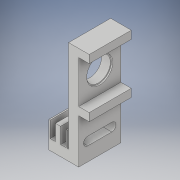
# Autodesk Inventor part: RotateLimitSwitchHolder
Saved by Autodesk Inventor 2018.3 (Build 223284000, 284)
## iProperties
Created: 2019-09-02
Part Number: RotateLimitSwitchHolder
Material: Generic
Document SubType Name: Modeling
Designer: Srinity
Density: 1 g/cm^3
Appearance: Default
Author: Srinity
Autodesk Inventor part; units mm, degrees
ref_plane "YZ Plane" through (0, 0, 0) normal (1, 0, 0) x (0, 1, 0)
ref_plane "XZ Plane" through (0, 0, 0) normal (0, 1, 0) x (-1, 0, 0)
ref_plane "XY Plane" through (0, 0, 0) normal (0, 0, 1) x (1, 0, 0)
sketch "Sketch1" plane through (0, 0, 0) normal (0, 0, 1) x (1, 0, 0)
  line L0 (10.0241, 19.7036) -> (11.6941, 19.7036)
  line L1 (11.6941, 19.7036) -> (11.6941, -12.0464)
  line L2 (11.6941, -12.0464) -> (10.0241, -12.0464)
  line L3 (10.0241, -12.0464) -> (10.0241, 19.7036)
  line L4 (11.6941, -5.6964) -> (18.1941, -5.6964)
  line L5 (18.1941, -5.6964) -> (18.1941, -12.0464)
  line L6 (18.1941, -12.0464) -> (11.6941, -12.0464)
  line L7 (11.6941, -12.0464) -> (11.6941, -5.6964)
  line L8 (18.1941, 19.7036) -> (24.3941, 19.7036)
  line L9 (24.3941, 19.7036) -> (24.3941, -12.0464)
  line L10 (24.3941, -12.0464) -> (18.1941, -12.0464)
  line L11 (18.1941, -12.0464) -> (18.1941, 19.7036)
  line L12 (24.3941, -5.6964) -> (30.8941, -5.6964)
  line L13 (30.8941, -5.6964) -> (30.8941, -12.0464)
  line L14 (30.8941, -12.0464) -> (24.3941, -12.0464)
  line L15 (24.3941, -12.0464) -> (24.3941, -5.6964)
  line L16 (30.8941, 19.7036) -> (32.5641, 19.7036)
  line L17 (32.5641, 19.7036) -> (32.5641, -12.0464)
  line L18 (32.5641, -12.0464) -> (30.8941, -12.0464)
  line L19 (30.8941, -12.0464) -> (30.8941, 19.7036)
  line L20 (14.9441, -5.6964) -> (14.9441, -6.8027)
  line L21 (27.6441, -5.6964) -> (27.6441, -11.0357)
  line L22 (10.0241, 0.6536) -> (32.5641, 0.6536)
  line L23 (32.5641, 0.6536) -> (32.5641, -12.0464)
  line L24 (32.5641, -12.0464) -> (10.0241, -12.0464)
  line L25 (10.0241, -12.0464) -> (10.0241, 0.6536)
  line L26 (32.5641, -12.0464) -> (46.1861, -12.0464)
  line L27 (46.1861, -12.0464) -> (46.1861, 0.6536)
  line L28 (46.1861, 0.6536) -> (32.5641, 0.6536)
  line L29 (32.5641, 0.6536) -> (32.5641, -12.0464)
  line L30 (33.9941, 0.6536) -> (46.1861, 0.6536)
  line L31 (46.1861, 0.6536) -> (46.1861, 111.9786)
  line L32 (46.1861, 111.9786) -> (33.9941, 111.9786)
  line L33 (33.9941, 111.9786) -> (33.9941, 0.6536)
  line L34 (46.1861, 41.7286) -> (58.8861, 41.7286)
  line L35 (58.8861, 41.7286) -> (58.8861, 51.2536)
  line L36 (58.8861, 51.2536) -> (46.1861, 51.2536)
  line L37 (46.1861, 51.2536) -> (46.1861, 41.7286)
  line L38 (46.1861, 102.4536) -> (58.8861, 102.4536)
  line L39 (58.8861, 102.4536) -> (58.8861, 111.9786)
  line L40 (58.8861, 111.9786) -> (46.1861, 111.9786)
  line L41 (46.1861, 111.9786) -> (46.1861, 102.4536)
  line L42 (-51.3447, 76.8536) -> (150.8271, 76.8536) construction
  point P0 (0, 0)
  dimension "d0" = 6.5
  dimension "d1" = 6.5
  dimension "d4" = 12.7
  dimension "d5" = 1.67
  dimension "d6" = 25.4
  dimension "d51" = 9.525
  dimension "d52" = 9.525
  dimension "d53" = 51.2
  dimension "d54" = 57.15
  dimension "d55" = 25.6
  dimension "d57" = 12.7
  dimension "d58" = 12.192
  dimension "d59" = 18.542
  dimension "d60" = 12.7
  dimension "d86" = 76.2
  constraints: 86 end point, 20 collinear, 20 parallel, 11 horizontal, 10 perpendicular, 4 point on line, 2 midpoint, 2 vertical
  measures "d0" distance between parallel lines of L11 L1
  measures "d1" distance between parallel lines of L19 L9
  measures "d4" distance between parallel lines of L21 L20
  measures "d5" distance of L0.start L0.end
  measures "d6" distance between parallel lines of L4 L8
  measures "d51" distance of L34.end L35.end
  measures "d52" distance of L38.end L39.end
  measures "d53" distance between parallel lines of L38 L36
  measures "d54" distance between parallel lines of L8 L42
  measures "d55" distance between parallel lines of L42 L36
  measures "d57" distance of L34.start L34.end
  measures "d58" distance of L31.end L32.end
  measures "d59" distance between parallel lines of L21 L31
  measures "d60" distance of L28.end L26.start
  measures "d86" distance between parallel lines of L28 L42
extrude "Extrusion1" add sketch "Sketch1" along normal blind 50.8
sketch "Sketch9" plane through (46.1861, 51.2536, 0) normal (1, 0, 0) x (0, 0, -1)
  circle A0 centre (-25.4, 25.6) radius 15.7575
  line L0 (0, 0) -> (0, 51.2) projected
  line L1 (0, 51.2) -> (-50.8, 51.2) projected
  point P0 (0, -51.2536)
  dimension "d61" = 31.515
  dimension "d62" = 25.4
  dimension "d63" = 25.6
  constraints: 1 centre point
  measures "d61" diameter of A0
  measures "d62" distance from line of A0.centre L0
  measures "d63" distance from line of A0.centre L1
extrude "Extrusion8" cut sketch "Sketch9" against normal blind 1.651
sketch "Sketch10" plane through (44.5351, 76.8536, 25.4) normal (1, 0, 0) x (0, 0, -1)
  circle A0 centre (0, 0) radius 15.7575 projected
  circle A1 centre (0, 0) radius 14.4875
  point P0 (25.4, -76.8536)
  dimension "d66" = 28.975
  constraints: 1 centre point, 1 coincident
  measures "d66" diameter of A1
extrude "Extrusion9" cut sketch "Sketch10" against normal through all contours A1
sketch "Sketch11" plane through (10.0241, -12.0464, 0) normal (-1, 0, 0) x (0, 0, 1)
  circle A0 centre (25.4, 36.35) radius 2.25
  line L0 (0, 124.025) -> (0, 12.7) projected
  circle A1 centre (10.9, 21.85) radius 1.3
  circle A2 centre (20.4, 21.85) radius 1.3
  circle A3 centre (30.4, 21.85) radius 1.3
  circle A4 centre (39.9, 21.85) radius 1.3
  circle A5 centre (25.4, 88.9) radius 14.4875 projected
  line L1 (36.7449, 38.6) -> (7.7398, 38.6) construction
  point P0 (0, 12.0464)
  dimension "d69" = 4.5
  dimension "d70" = 25.4
  dimension "d71" = 9.5
  dimension "d72" = 9.5
  dimension "d73" = 2.6
  dimension "d74" = 14.5
  dimension "d75" = 50.3
  dimension "d76" = 14.5
  dimension "d77" = 14.5
  constraints: 5 centre point, 3 equal radius, 3 horizontal alignment, 2 end point, 1 horizontal, 1 tangent
  measures "d69" diameter of A0
  measures "d70" distance from line of A0.centre L0
  measures "d71" distance of A2.centre A1.centre
  measures "d72" distance of A3.centre A4.centre
  measures "d73" diameter of A4
  measures "d74" vertical distance of A2.centre A0.centre
  measures "d75" distance from line of A5.centre L1
  measures "d76" horizontal distance of A1.centre A0.centre
  measures "d77" horizontal distance of A0.centre A4.centre
extrude "Extrusion10" cut sketch "Sketch11" against normal through all contours A1 | A2 | A3 | A4
sketch "Sketch14" plane through (30.8941, 0.6536, 0) normal (-1, 0, 0) x (0, 0, 1)
  circle A0 centre (39.9, 9.15) radius 1.3 projected
  arc A1 (39.9, 4.705) -> (39.9, 13.595) centre (39.9, 9.15) ccw
  circle A2 centre (30.4, 9.15) radius 1.3 projected
  arc A3 (30.4, 13.595) -> (30.4, 4.705) centre (30.4, 9.15) ccw
  line L0 (39.9, 4.705) -> (30.4, 4.705)
  line L1 (39.9, 13.595) -> (30.4, 13.595)
  arc A4 (39.9, 13.595) -> (39.9, 4.705) centre (39.9, 9.15) ccw
  arc A5 (30.4, 4.705) -> (30.4, 13.595) centre (30.4, 9.15) ccw
  point P0 (0, -0.6536)
  dimension "d87" = 8.89
  constraints: 8 point on circle, 4 centre point, 4 end point, 2 coincident, 2 tangent, 1 equal radius, 1 parallel
  measures "d87" diameter of A1
extrude "Extrusion13" cut sketch "Sketch14" against normal up to surface (1.67 mm away)
sketch "Sketch15" plane through (10.0241, -12.0464, 0) normal (-1, 0, 0) x (0, 0, 1)
  circle A0 centre (20.4, 21.85) radius 1.3 projected
  arc A1 (20.4, 17.405) -> (20.4, 26.295) centre (20.4, 21.85) ccw
  circle A2 centre (10.9, 21.85) radius 1.3 projected
  arc A3 (10.9, 26.295) -> (10.9, 17.405) centre (10.9, 21.85) ccw
  line L0 (20.4, 17.405) -> (10.9, 17.405)
  line L1 (10.9, 26.295) -> (20.4, 26.295)
  arc A4 (20.4, 26.295) -> (20.4, 17.405) centre (20.4, 21.85) ccw
  arc A5 (10.9, 17.405) -> (10.9, 26.295) centre (10.9, 21.85) ccw
  point P0 (0, 12.0464)
  dimension "d90" = 8.89
  constraints: 8 point on circle, 4 centre point, 4 end point, 2 coincident, 2 tangent, 1 equal radius, 1 parallel
  measures "d90" diameter of A1
extrude "Extrusion14" cut sketch "Sketch15" against normal up to surface (1.67 mm away)
sketch "Sketch16" plane through (46.1861, -12.0464, 0) normal (1, 0, 0) x (0, 0, -1)
  circle A0 centre (-10.9, 21.85) radius 1.3 projected
  arc A1 (-10.9, 16.77) -> (-10.9, 26.93) centre (-10.9, 21.85) ccw
  circle A2 centre (-39.9, 21.85) radius 1.3 projected
  arc A3 (-39.9, 26.93) -> (-39.9, 16.77) centre (-39.9, 21.85) ccw
  line L0 (-10.9, 16.77) -> (-39.9, 16.77)
  line L1 (-39.9, 26.93) -> (-10.9, 26.93)
  arc A4 (-10.9, 26.93) -> (-10.9, 16.77) centre (-10.9, 21.85) ccw
  arc A5 (-39.9, 16.77) -> (-39.9, 26.93) centre (-39.9, 21.85) ccw
  point P0 (0, 12.0464)
  dimension "d93" = 10.16
  constraints: 8 point on circle, 4 centre point, 4 end point, 2 coincident, 1 equal radius, 1 horizontal, 1 parallel, 1 tangent
  measures "d93" diameter of A1
extrude "Extrusion15" cut sketch "Sketch16" against normal up to surface (12.192 mm away)
sketch "Sketch17" plane through (24.3941, 0.6536, 0) normal (0, 1, 0) x (1, 0, 0)
  line L0 (6.5, -34.925) -> (0, -34.925)
  line L1 (0, -34.925) -> (0, -15.875)
  line L2 (0, -15.875) -> (6.5, -15.875)
  line L3 (6.5, -15.875) -> (6.5, -34.925)
  line L4 (-6.2, -34.925) -> (-12.7, -34.925)
  line L5 (-12.7, -34.925) -> (-12.7, -15.875)
  line L6 (-12.7, -15.875) -> (-6.2, -15.875)
  line L7 (-6.2, -15.875) -> (-6.2, -34.925)
  line L8 (6.5, -25.4) -> (0, -25.4) construction
  line L9 (0, 0) -> (6.5, 0) projected
  line L10 (6.5, 0) -> (6.5, -50.8) projected
  line L11 (0, 0) -> (0, -50.8) projected
  line L12 (-6.2, 0) -> (-6.2, -50.8) projected
  line L13 (-12.7, 0) -> (-12.7, -50.8) projected
  point P0 (-24.3941, 0)
  dimension "d96" = 19.05
  dimension "d97" = 25.4
  constraints: 18 end point, 6 collinear, 4 parallel, 2 horizontal, 2 midpoint, 2 perpendicular
  measures "d96" distance of L0.end L1.end
  measures "d97" distance between parallel lines of L8 L9
extrude "Extrusion16" cut sketch "Sketch17" against normal through all contours L0 L1 L2 L3 | L4 L5 L6 L7
equation "\"d0\" = d1"
equation "\"d55\" = 0.5 * d53"
equation "\"d63\" = d55"
equation "\"d72\" = d71"
equation "\"d77\" = d76"
equation "\"d91\" = d90"
body "Solid1"
